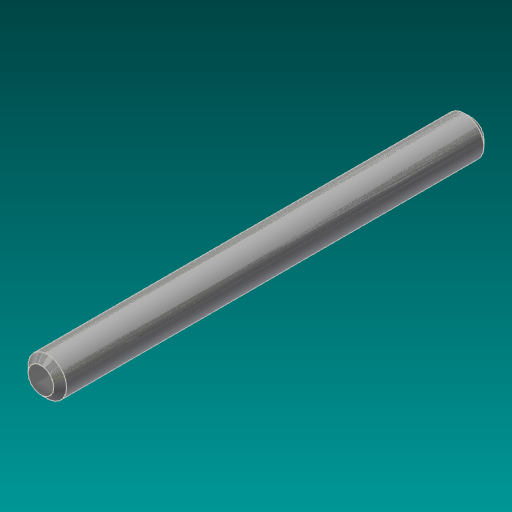
# Autodesk Inventor part: A1-19037-300-07 Trap rod
Saved by Autodesk Inventor 2017.3 (Build 213256000, 256)
## iProperties
Created: 2017-11-23
Part Number: A1-19037-300-07 Trap rod
Material: Steel, Mild
Document SubType Name: Modeling
Designer: Graeme_Van_Dongen
Density: 7.85 g/cm^3
Appearance: Steel
Description: Ø3/8" x 4 9/16" ROUND BAR, A36
Mass: 58.9685 g
Surface Area: 32.6305 cm^2
Volume: 7.51191 cm^3
Project: A1-19037--CNUL Albian CST laterals
Constructed By: Graeme_Van_Dongen
Project Name: CST laterals
Author: Graeme_Van_Dongen
Autodesk Inventor part; units mm, degrees
ref_plane "YZ Plane" through (0, 0, 0) normal (1, 0, 0) x (0, 1, 0)
ref_plane "XZ Plane" through (0, 0, 0) normal (0, 1, 0) x (-1, 0, 0)
ref_plane "XY Plane" through (0, 0, 0) normal (0, 0, 1) x (1, 0, 0)
sketch "Sketch1" plane through (0, 0, 0) normal (0, 0, 1) x (1, 0, 0)
  circle A0 centre (0, 0) radius 4.7625
  dimension "d0" = 9.525
  constraints: 1 centre point, 1 coincident
  measures "d0" diameter of A0
extrude "Extrusion1" add sketch "Sketch1" along normal blind 106.3625
chamfer "Chamfer1" distance 1.5875 angle 45 2 edges at (-4.7625, 0, 0) (-4.7625, 0, 106.3625)
body "Solid1"
